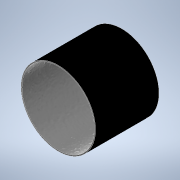
# Autodesk Inventor part: velcro
Saved by Autodesk Inventor 2022 (Build 260153000, 153)
## iProperties
Created: 2024-02-25
Part Number: velcro
Material: Genérico
Document SubType Name: Modeling
Designer: Daniel
Density: 1 g/cm^3
Appearance: Texturizado fino - Preto
Author: Daniel
Autodesk Inventor part; units mm, degrees
ref_plane "YZ Plane" through (0, 0, 0) normal (1, 0, 0) x (0, 1, 0)
ref_plane "XZ Plane" through (0, 0, 0) normal (0, 1, 0) x (-1, 0, 0)
ref_plane "XY Plane" through (0, 0, 0) normal (0, 0, 1) x (1, 0, 0)
sketch "Esboço1" plane through (0, 0, 0) normal (0, 0, 1) x (1, 0, 0)
  circle A0 centre (0, 0) radius 28.6624
  circle A1 centre (0, 0) radius 29.4124
  dimension "d0" = 57.3248
  dimension "d1" = 0.75
  constraints: 2 centre point, 1 coincident
  measures "d0" diameter of A0
  measures "d1" radial gap between concentric circles of A0 A1
extrude "Extrusão1" add sketch "Esboço1" along normal blind 50
